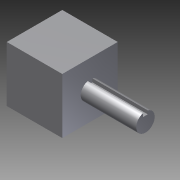
# Autodesk Inventor part: BaneBots P60 4 to1 gearbox
Saved by Autodesk Inventor 2011 SP1 (Build 150282100, 282)
## iProperties
Created: 2013-01-16
Part Number: BaneBots P60 4 to1 gearbox
Document SubType Name: Modeling
Designer: 961407
Density: 1 g/cm^3
Author: 961407
Autodesk Inventor part; units mm, degrees
ref_plane "YZ Plane" through (0, 0, 0) normal (1, 0, 0) x (0, 1, 0)
ref_plane "XZ Plane" through (0, 0, 0) normal (0, 1, 0) x (-1, 0, 0)
ref_plane "XY Plane" through (0, 0, 0) normal (0, 0, 1) x (1, 0, 0)
sketch "Sketch1" plane through (0, 0, 0) normal (0, 0, 1) x (1, 0, 0)
  line L0 (-38.1, 0) -> (0, 0)
  line L1 (0, 0) -> (0, 38.1)
  line L2 (0, 38.1) -> (-38.1, 38.1)
  line L3 (-38.1, 38.1) -> (-38.1, 0)
  dimension "d0" = 38.1
  dimension "d1" = 38.1
  constraints: 8 end point, 2 parallel, 1 horizontal, 1 perpendicular
  measures "d0" distance of L0.end L1.end
  measures "d1" distance of L0.start L0.end
extrude "Extrusion1" add sketch "Sketch1" along normal blind 38.1
sketch "Sketch2" plane through (0, 0, 0) normal (1, 0, 0) x (0, 0, -1)
  line L0 (-38.1, 38.1) -> (-38.1, 0) projected
  line L1 (0, 0) -> (-38.1, 0) projected
  line L2 (0, 0) -> (0, 38.1) projected
  line L3 (0, 38.1) -> (-38.1, 38.1) projected
  line L4 (-38.1, 38.1) -> (-38.1, 0) projected
  line L5 (0, 0) -> (-38.1, 0) projected
  line L6 (0, 0) -> (0, 38.1) projected
  line L7 (0, 38.1) -> (-38.1, 38.1) projected
  circle A0 centre (-19.05, 19.05) radius 6.35
  dimension "d4" = 19.05
  dimension "d5" = 12.7
  constraints: 1 centre point
  measures "d4" distance from line of L2 A0.centre
  measures "d5" diameter of A0
sketch "Sketch3" plane through (0, 0, 0) normal (1, 0, 0) x (0, 0, -1)
  line L0 (0, 38.1) -> (-38.1, 38.1) projected
  circle A0 centre (-19.05, 19.05) radius 6.35 projected
  line L1 (-20.6502, 25.1951) -> (-20.6502, 22.86)
  line L2 (-20.6502, 22.86) -> (-17.4752, 22.86)
  line L3 (-17.4752, 22.86) -> (-17.4752, 25.2016)
  point P0 (-19.05, 25.4)
  dimension "d6" = 1.6002
  dimension "d7" = 3.175
  dimension "d8" = 1.6002
  dimension "d9" = 2.54
  constraints: 6 end point, 3 point on circle, 2 perpendicular, 1 parallel
  measures "d6" distance from line of L1 A0.centre
  measures "d7" distance between parallel lines of L3 L1
  measures "d8" distance from line of L1 point (-19.05, 25.4)
  measures "d9" distance from line of L2 point (-19.05, 25.4)
extrude "Extrusion2" add sketch "Sketch3" along normal blind 38.1 contours A0 L1 L2 L3 picked at (-18.8789, 19.481)
sketch "Sketch4" plane through (-38.1, 0, 0) normal (-1, 0, 0) x (0, 0, 1)
  line L0 (38.1, 0) -> (38.1, 38.1) projected
  line L1 (0, 0) -> (38.1, 0) projected
  circle A0 centre (19.05, 19.05) radius 2.6035
  dimension "d12" = 19.05
  dimension "d13" = 19.05
  dimension "d14" = 5.207
  constraints: 1 centre point
  measures "d12" distance from line of L0 A0.centre
  measures "d13" distance from line of L1 A0.centre
  measures "d14" diameter of A0
extrude "Extrusion3" cut sketch "Sketch4" against normal blind 7.747
body "Solid1"
